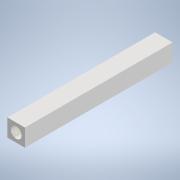
# Autodesk Inventor part: plunger
Saved by Autodesk Inventor 2021 (Build 250183000, 183)
## iProperties
Created: 2021-08-22
Part Number: plunger
Material: Generic
Document SubType Name: Modeling
Designer: techv
Density: 1 g/cm^3
Appearance: Default
Author: techv
Autodesk Inventor part; units mm, degrees
ref_plane "YZ Plane" through (0, 0, 0) normal (1, 0, 0) x (0, 1, 0)
ref_plane "XZ Plane" through (0, 0, 0) normal (0, 1, 0) x (-1, 0, 0)
ref_plane "XY Plane" through (0, 0, 0) normal (0, 0, 1) x (1, 0, 0)
sketch "Sketch1" plane through (0, 0, 0) normal (0, 0, 1) x (1, 0, 0)
  line L0 (5, -5) -> (5, 5) projected
  line L1 (-5, -5) -> (5, -5) projected
  line L2 (-5, 5) -> (-5, -5) projected
  line L3 (5, 5) -> (-5, 5) projected
  circle A0 centre (0, 0) radius 3
  line L4 (2.8868, -5) -> (5.7735, 0) projected
  line L5 (2.8868, -5) -> (5.7735, 0) projected
  line L6 (-2.8868, -5) -> (2.8868, -5) projected
  line L7 (-5.7735, 0) -> (-2.8868, -5) projected
  line L8 (-2.8868, 5) -> (-5.7735, 0) projected
  line L9 (2.8868, 5) -> (-2.8868, 5) projected
  line L10 (5.7735, 0) -> (2.8868, 5) projected
  circle A1 centre (0, 0) radius 2.9998 projected
  line L11 (6.5, -6.5) -> (-6.5, -6.5)
  line L12 (-6.5, -6.5) -> (-6.5, 6.5)
  line L13 (-6.5, 6.5) -> (6.5, 6.5)
  line L14 (6.5, 6.5) -> (6.5, -6.5)
  line L15 (6.5, -6.5) -> (-6.5, 6.5) construction
  line L16 (-6.5, -6.5) -> (6.5, 6.5) construction
  dimension "d0" = 6
  dimension "d7" = 13
  dimension "d8" = 13
  constraints: 12 end point, 2 midpoint, 2 parallel, 1 centre point, 1 coincident, 1 horizontal, 1 perpendicular, 2 other
  measures "d0" diameter of A0
  measures "d7" distance of L12.end L13.end
  measures "d8" distance of L11.end L12.end
extrude "Extrusion1" add sketch "Sketch1" along normal blind 110 contours L1 L4 L0 | L4 L1 L7 L2 L8 L3 L10 L0 | L0 L10 L4 | L10 L3 L0 | L1 L2 L7 | L7 L8 L2 | L8 L2 L3 | A0 | L11 L12 L13 L14
sketch "Sketch2" plane through (0, 0, 110) normal (0, 0, 1) x (1, 0, 0)
  point P0 (0, 0)
sketch "Sketch3" plane through (0, 0, 110) normal (0, 0, 1) x (1, 0, 0)
  circle A0 centre (0, 0) radius 4
  circle A1 centre (0, 0) radius 3
  line L0 (2.8868, -5) -> (5.7735, 0)
  line L1 (5.7735, 0) -> (2.8868, 5)
  line L2 (2.8868, 5) -> (-2.8868, 5)
  line L3 (-2.8868, 5) -> (-5.7735, 0)
  line L4 (-5.7735, 0) -> (-2.8868, -5)
  line L5 (-2.8868, -5) -> (2.8868, -5)
extrude "Extrusion2" cut sketch "Sketch3" against normal blind 3.22 contours A0 | A1 | L5 L4 L3 L2 L1 L0
sketch "Sketch4" plane through (0, 0, 0) normal (0, 0, -1) x (-1, 0, 0)
  circle A0 centre (0, 0) radius 3.5
  dimension "d9" = 7
  constraints: 1 centre point, 1 coincident
  measures "d9" diameter of A0
extrude "Extrusion3" cut sketch "Sketch4" against normal through all
body "Solid1"
